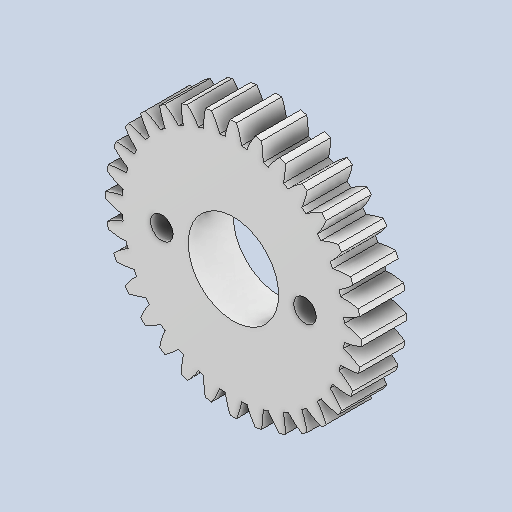
# Autodesk Inventor part: 平歯車1
Saved by Autodesk Inventor 2025.2 (Build 292293000, 293)
## iProperties
CustomPartVersion: 1
Created: 2025-01-07
Part Number: 平歯車1
Material: ABS プラスチック
Document SubType Name: Modeling
Designer: haruy
Categories: <?xml version="1.0" encoding="UTF-16"?> <MemberInstance><Categories><FamilyTemplate><FamilyTemplateParameter ValueType="xs:double" Id="1" ObjectReferenceKey="da_z" ObjectType="kUserParameterObject"/><FamilyTemplateParameter ValueType="xs:double" Id="2" ObjectReferenceKey="da_b" ObjectType="kUserParameterObject"/><FamilyTemplateParameter ValueType="xs:double" Id="3" ObjectReferenceKey="da_beta" ObjectType="kUserParameterObject"/><FamilyTemplateParameter ValueType="xs:double" Id="4" ObjectReferenceKey="da_da" ObjectType="kUserParameterObject"/><FamilyTemplateParameter ValueType="xs:double" Id="5" ObjectReferenceKey="da_aw" ObjectType="kUserParameterObject"/><FamilyTemplateParameter ValueType="xs:string" Id="6" ObjectReferenceKey="EAIAABAAAACIAQAAAAAAAIAAAAAAAAAA" ObjectType="83910656" SubObjectId="SurfaceGeometry"/></FamilyTemplate><ParamToTemplateMap><ParamToTemplate CategoryParameter="//CategoryParameter[@InternalName='046C89C9-8512-4d59-83FE-43B91F4F132A']" TemplateParameter="1"/><ParamToTemplate CategoryParameter="//CategoryParameter[@InternalName='2552DF32-E462-4b46-AEBF-C6C7768E72AC']" TemplateParameter="2"/><ParamToTemplate CategoryParameter="//CategoryParameter[@InternalName='C9EE641D-15FC-4fae-A226-E94C4372FDD7']" TemplateParameter="3"/><ParamToTemplate><ParamToTemplate CategoryParameter="//CategoryParameter[@InternalName='00B6519A-459B-49c7-AD84-2E56D39A5744']" ConstantValue="0.000000"/></ParamToTemplate><ParamToTemplate><ParamToTemplate CategoryParameter="//CategoryParameter[@InternalName='04B31F0E-C7A6-4894-AA32-9629BEFACF47']" ConstantValue="1.000000"/></ParamToTemplate><ParamToTemplate><ParamToTemplate CategoryParameter="//CategoryParameter[@InternalName='43CBEC2E-7847-49e7-A936-2F7889FCB2D9']" ConstantValue="0.250000"/></ParamToTemplate><ParamToTemplate><ParamToTemplate CategoryParameter="//CategoryParameter[@InternalName='B1EFC894-105D-4ebd-86BF-FA20ED196853']" ConstantValue="0.350000"/></ParamToTemplate><ParamToTemplate><ParamToTemplate CategoryParameter="//CategoryParameter[@InternalName='51175063-3D10-4879-93E8-6246FE8B403D']" ConstantValue="2060000000.000000"/></ParamToTemplate><ParamToTemplate><ParamToTemplate CategoryParameter="//CategoryParameter[@InternalName='A3A52E27-4454-46a9-B0BD-C932399B70AF']" ConstantValue="0.300000"/></ParamToTemplate><ParamToTemplate><ParamToTemplate CategoryParameter="//CategoryParameter[@InternalName='91B76062-C214-41d9-B1B9-14D2AB99603D']" ConstantValue="0.100000"/></ParamToTemplate><ParamToTemplate><ParamToTemplate CategoryParameter="//CategoryParameter[@InternalName='374E806E-8B8A-4dda-A9AA-1039D6500AD2']" ConstantValue="10.000000"/></ParamToTemplate><ParamToTemplate><ParamToTemplate CategoryParameter="//CategoryParameter[@InternalName='2D373A89-B862-43d6-8D0B-0CBF12AB9F6C']" ConstantValue="0.349066"/></ParamToTemplate><ParamToTemplate CategoryParameter="//CategoryParameter[@InternalName='37777632-D6A2-4fac-9D53-DB8ACD95C989']" TemplateParameter="4"/><ParamToTemplate CategoryParameter="//CategoryParameter[@InternalName='FD1017F1-B727-4f7e-9707-0F86F1FF9423']" TemplateParameter="5"/><ParamToTemplate><ParamToTemplate CategoryParameter="//CategoryParameter[@InternalName='9E1B4470-B2D3-4ff1-B813-535BB4CDF51A']" ConstantValue="3520000.000000"/></ParamToTemplate><ParamToTemplate><ParamToTemplate CategoryParameter="//CategoryParameter[@InternalName='F8452263-BFF6-458c-9FB1-07C4B99E95CD']" ConstantValue="11400000.000000"/></ParamToTemplate><ParamToTemplate><ParamToTemplate CategoryParameter="//CategoryParameter[@InternalName='3E3BB259-FD49-497f-8171-6EBC954A3479']" ConstantValue="2.000000"/></ParamToTemplate><ParamToTemplate CategoryParameter="//CategoryParameter[@InternalName='27C3BAF2-7550-4e4b-AE2C-0DB134B7D9B7']" TemplateParameter="6"/></ParamToTemplateMap><Category DisplayName="Gear" InternalName="DC85795E-93AB-48d5-8EEE-5A27447B64BD" Mnemonic="Gear"><CategoryParameter DisplayName="z" InternalName="046C89C9-8512-4d59-83FE-43B91F4F132A" Mnemonic="z"/><CategoryParameter DisplayName="b" InternalName="2552DF32-E462-4b46-AEBF-C6C7768E72AC" Mnemonic="b"/><CategoryParameter DisplayName="||b|" InternalName="C9EE641D-15FC-4fae-A226-E94C4372FDD7" Mnemonic="beta"/><CategoryParameter DisplayName="x" InternalName="00B6519A-459B-49c7-AD84-2E56D39A5744" Mnemonic="x"/><CategoryParameter DisplayName="a*" InternalName="04B31F0E-C7A6-4894-AA32-9629BEFACF47" Mnemonic="a"/><CategoryParameter DisplayName="c*" InternalName="43CBEC2E-7847-49e7-A936-2F7889FCB2D9" Mnemonic="c"/><CategoryParameter DisplayName="r|.f|*" InternalName="B1EFC894-105D-4ebd-86BF-FA20ED196853" Mnemonic="rf"/><CategoryParameter DisplayName="E" InternalName="51175063-3D10-4879-93E8-6246FE8B403D" Mnemonic="E"/><CategoryParameter DisplayName="||m|" InternalName="A3A52E27-4454-46a9-B0BD-C932399B70AF" Mnemonic="mi"/><Category DisplayName="SpurGear" InternalName="26C5A22E-A91E-4dfd-A3B3-23CCAFAE1764" Mnemonic="SpurGear"><CategoryParameter DisplayName="m" InternalName="91B76062-C214-41d9-B1B9-14D2AB99603D" Mnemonic="m"/><CategoryParameter DisplayName="P" InternalName="374E806E-8B8A-4dda-A9AA-1039D6500AD2" Mnemonic="PP"/><CategoryParameter DisplayName="||a|" InternalName="2D373A89-B862-43d6-8D0B-0CBF12AB9F6C" Mnemonic="alpha"/><CategoryParameter DisplayName="d|.a|" InternalName="37777632-D6A2-4fac-9D53-DB8ACD95C989" Mnemonic="da"/><CategoryParameter DisplayName="a|.w|" InternalName="FD1017F1-B727-4f7e-9707-0F86F1FF9423" Mnemonic="aw"/><CategoryParameter DisplayName="||s||.Flim|" InternalName="9E1B4470-B2D3-4ff1-B813-535BB4CDF51A" Mnemonic="sFlim"/><CategoryParameter DisplayName="||s||.Hlim|" InternalName="F8452263-BFF6-458c-9FB1-07C4B99E95CD" Mnemonic="sHlim"/><CategoryParameter DisplayName="タイプ" InternalName="3E3BB259-FD49-497f-8171-6EBC954A3479" Mnemonic="type"/><CategoryParameter DisplayName="PitchDiameter" InternalName="27C3BAF2-7550-4e4b-AE2C-0DB134B7D9B7" Mnemonic="IDS_PITCHDIAM"/></Category></Category></Categories></MemberInstance>
Density: 1.06 g/cm^3
Appearance: 滑らか - 白
Mass: 37.6143 g
Surface Area: 28.126 cm^2
Volume: 4.79163 cm^3
Author: haruy
Autodesk Inventor part; units mm, degrees
sketch "Sketch1" plane through (0, 0, 0) normal (0, 0, 1) x (1, 0, 0)
  circle A0 centre (0, 0) radius 17
  dimension "d0" = 34
  constraints: 1 centre point
  measures "d0" diameter of A0
extrude "Extrusion1" add sketch "Sketch1" along normal blind 6
ref_plane "Work Plane2" through (0, 0, 3) normal (0, 0, 1) x (1, 0, 0)
sketch "Sketch2" plane through (0, 0, 0) normal (0, 0, -1) x (-1, 0, 0)
  circle A0 centre (0, 0) radius 17 projected
  circle A1 centre (0, 0) radius 16
  dimension "d3" = 32
  constraints: 1 centre point, 1 coincident
  measures "d3" diameter of A1
surface extrude "ピッチ円直径" sketch "Sketch2" against normal through all shown no curves A1
ref_plane "Work Plane8" through (0, 0, 0) normal (0.9951847, 0.0980171, 0) x (0, 0, 1)
ref_plane "Work Plane9" through (0, 0, 0) normal (1, 0, 0) x (0, 1, 0)
spur gear teeth "平歯車" teeth 32 pitch diameter 32 tip diameter 34 root diameter 29.5 face width 6 start plane through (0, 0, 0) normal (0, 0, -1) x (-1, 0, 0)
sketch "スケッチ3" plane through (0, 0, 6) normal (0, 0, 1) x (1, 0, 0)
  circle A0 centre (0, 0) radius 6
  circle A1 centre (0, 0) radius 9.5
  circle A2 centre (-9.5, 0) radius 1.5
  circle A3 centre (9.5, 0) radius 1.5
  dimension "d50" = 19
  dimension "d49" = 12
  dimension "d51" = 3
  dimension "d54" = 360
  constraints: 3 centre point, 2 coincident, 1 horizontal alignment, 7 other
  measures "d49" diameter of A0
  measures "d51" diameter of A2
extrude "押し出し2" cut sketch "スケッチ3" against normal blind 10 contours A0 | A1 A3 | A1 A3 | A2 A1 | A1 A2
sketch "スケッチ4" plane through (0, 0, 6) normal (0, 0, 1) x (1, 0, 0)
  circle A0 centre (9.5, 0) radius 1.5 projected
  circle A1 centre (-9.5, 0) radius 1.5 projected
  circle A2 centre (0, 0) radius 6 projected
  arc A3 (-3.7247, 16.5869) -> (-3.934, 14.2157) centre (6.3329, 14.5044) ccw projected
  arc A4 (-3.934, 14.2157) -> (-4.6268, 14.0055) centre (0, 0) ccw projected
  arc A5 (-4.6268, 14.0055) -> (-6.1182, 15.8609) centre (-13.3238, 8.5416) ccw projected
  arc A6 (-6.1182, 15.8609) -> (-6.8891, 15.5416) centre (0, 0) ccw projected
  arc A7 (-6.8891, 15.5416) -> (-6.6318, 13.1751) centre (3.3815, 15.4612) ccw projected
  arc A8 (-6.6318, 13.1751) -> (-7.2702, 12.8338) centre (0, 0) ccw projected
  arc A9 (-7.2702, 12.8338) -> (-9.095, 14.3625) centre (-14.7342, 5.7781) ccw projected
  arc A10 (-9.095, 14.3625) -> (-9.7887, 13.8989) centre (0, 0) ccw projected
  arc A11 (-9.7887, 13.8989) -> (-9.0747, 11.6281) centre (0.3002, 15.8238) ccw projected
  arc A12 (-9.0747, 11.6281) -> (-9.6343, 11.1688) centre (0, 0) ccw projected
  arc A13 (-9.6343, 11.1688) -> (-11.7222, 12.3122) centre (-15.5783, 2.7926) ccw projected
  arc A14 (-11.7222, 12.3122) -> (-12.3122, 11.7222) centre (0, 0) ccw projected
  arc A15 (-12.3122, 11.7222) -> (-11.1688, 9.6343) centre (-2.7926, 15.5783) ccw projected
  arc A16 (-11.1688, 9.6343) -> (-11.6281, 9.0747) centre (0, 0) ccw projected
  arc A17 (-11.6281, 9.0747) -> (-13.8989, 9.7887) centre (-15.8238, -0.3002) ccw projected
  arc A18 (-13.8989, 9.7887) -> (-14.3625, 9.095) centre (0, 0) ccw projected
  arc A19 (-14.3625, 9.095) -> (-12.8338, 7.2702) centre (-5.7781, 14.7342) ccw projected
  arc A20 (-12.8338, 7.2702) -> (-13.1751, 6.6318) centre (0, 0) ccw projected
  arc A21 (-13.1751, 6.6318) -> (-15.5416, 6.8891) centre (-15.4612, -3.3815) ccw projected
  arc A22 (-15.5416, 6.8891) -> (-15.8609, 6.1182) centre (0, 0) ccw projected
  arc A23 (-15.8609, 6.1182) -> (-14.0055, 4.6268) centre (-8.5416, 13.3238) ccw projected
  arc A24 (-14.0055, 4.6268) -> (-14.2157, 3.934) centre (0, 0) ccw projected
  arc A25 (-14.2157, 3.934) -> (-16.5869, 3.7247) centre (-14.5044, -6.3329) ccw projected
  arc A26 (-16.5869, 3.7247) -> (-16.7497, 2.9064) centre (0, 0) ccw projected
  arc A27 (-16.7497, 2.9064) -> (-14.6391, 1.8056) centre (-10.9768, 11.4014) ccw projected
  arc A28 (-14.6391, 1.8056) -> (-14.71, 1.0851) centre (0, 0) ccw projected
  arc A29 (-14.71, 1.0851) -> (-16.9949, 0.4172) centre (-12.9902, -9.0408) ccw projected
  arc A30 (-16.9949, 0.4172) -> (-16.9949, -0.4172) centre (0, 0) ccw projected
  arc A31 (-16.9949, -0.4172) -> (-14.71, -1.0851) centre (-12.9902, 9.0408) ccw projected
  arc A32 (-14.71, -1.0851) -> (-14.6391, -1.8056) centre (0, 0) ccw projected
  arc A33 (-14.6391, -1.8056) -> (-16.7497, -2.9064) centre (-10.9768, -11.4014) ccw projected
  arc A34 (-16.7497, -2.9064) -> (-16.5869, -3.7247) centre (0, 0) ccw projected
  arc A35 (-16.5869, -3.7247) -> (-14.2157, -3.934) centre (-14.5044, 6.3329) ccw projected
  arc A36 (-14.2157, -3.934) -> (-14.0055, -4.6268) centre (0, 0) ccw projected
  arc A37 (-14.0055, -4.6268) -> (-15.8609, -6.1182) centre (-8.5416, -13.3238) ccw projected
  arc A38 (-15.8609, -6.1182) -> (-15.5416, -6.8891) centre (0, 0) ccw projected
  arc A39 (-15.5416, -6.8891) -> (-13.1751, -6.6318) centre (-15.4612, 3.3815) ccw projected
  arc A40 (-13.1751, -6.6318) -> (-12.8338, -7.2702) centre (0, 0) ccw projected
  arc A41 (-12.8338, -7.2702) -> (-14.3625, -9.095) centre (-5.7781, -14.7342) ccw projected
  arc A42 (-14.3625, -9.095) -> (-13.8989, -9.7887) centre (0, 0) ccw projected
  arc A43 (-13.8989, -9.7887) -> (-11.6281, -9.0747) centre (-15.8238, 0.3002) ccw projected
  arc A44 (-11.6281, -9.0747) -> (-11.1688, -9.6343) centre (0, 0) ccw projected
  arc A45 (-11.1688, -9.6343) -> (-12.3122, -11.7222) centre (-2.7926, -15.5783) ccw projected
  arc A46 (-12.3122, -11.7222) -> (-11.7222, -12.3122) centre (0, 0) ccw projected
  arc A47 (-11.7222, -12.3122) -> (-9.6343, -11.1688) centre (-15.5783, -2.7926) ccw projected
  arc A48 (-9.6343, -11.1688) -> (-9.0747, -11.6281) centre (0, 0) ccw projected
  arc A49 (-9.0747, -11.6281) -> (-9.7887, -13.8989) centre (0.3002, -15.8238) ccw projected
  arc A50 (-9.7887, -13.8989) -> (-9.095, -14.3625) centre (0, 0) ccw projected
  arc A51 (-9.095, -14.3625) -> (-7.2702, -12.8338) centre (-14.7342, -5.7781) ccw projected
  arc A52 (-7.2702, -12.8338) -> (-6.6318, -13.1751) centre (0, 0) ccw projected
  arc A53 (-6.6318, -13.1751) -> (-6.8891, -15.5416) centre (3.3815, -15.4612) ccw projected
  arc A54 (-6.8891, -15.5416) -> (-6.1182, -15.8609) centre (0, 0) ccw projected
  arc A55 (-6.1182, -15.8609) -> (-4.6268, -14.0055) centre (-13.3238, -8.5416) ccw projected
  arc A56 (-4.6268, -14.0055) -> (-3.934, -14.2157) centre (0, 0) ccw projected
  arc A57 (-3.934, -14.2157) -> (-3.7247, -16.5869) centre (6.3329, -14.5044) ccw projected
  arc A58 (-3.7247, -16.5869) -> (-2.9064, -16.7497) centre (0, 0) ccw projected
  arc A59 (-2.9064, -16.7497) -> (-1.8056, -14.6391) centre (-11.4014, -10.9768) ccw projected
  arc A60 (-1.8056, -14.6391) -> (-1.0851, -14.71) centre (0, 0) ccw projected
  arc A61 (-1.0851, -14.71) -> (-0.4172, -16.9949) centre (9.0408, -12.9902) ccw projected
  arc A62 (-0.4172, -16.9949) -> (0.4172, -16.9949) centre (0, 0) ccw projected
  arc A63 (0.4172, -16.9949) -> (1.0851, -14.71) centre (-9.0408, -12.9902) ccw projected
  arc A64 (1.0851, -14.71) -> (1.8056, -14.6391) centre (0, 0) ccw projected
  arc A65 (1.8056, -14.6391) -> (2.9064, -16.7497) centre (11.4014, -10.9768) ccw projected
  arc A66 (2.9064, -16.7497) -> (3.7247, -16.5869) centre (0, 0) ccw projected
  arc A67 (3.7247, -16.5869) -> (3.934, -14.2157) centre (-6.3329, -14.5044) ccw projected
  arc A68 (3.934, -14.2157) -> (4.6268, -14.0055) centre (0, 0) ccw projected
  arc A69 (4.6268, -14.0055) -> (6.1182, -15.8609) centre (13.3238, -8.5416) ccw projected
  arc A70 (6.1182, -15.8609) -> (6.8891, -15.5416) centre (0, 0) ccw projected
  arc A71 (6.8891, -15.5416) -> (6.6318, -13.1751) centre (-3.3815, -15.4612) ccw projected
  arc A72 (6.6318, -13.1751) -> (7.2702, -12.8338) centre (0, 0) ccw projected
  arc A73 (7.2702, -12.8338) -> (9.095, -14.3625) centre (14.7342, -5.7781) ccw projected
  arc A74 (9.095, -14.3625) -> (9.7887, -13.8989) centre (0, 0) ccw projected
  arc A75 (9.7887, -13.8989) -> (9.0747, -11.6281) centre (-0.3002, -15.8238) ccw projected
  arc A76 (9.0747, -11.6281) -> (9.6343, -11.1688) centre (0, 0) ccw projected
  arc A77 (9.6343, -11.1688) -> (11.7222, -12.3122) centre (15.5783, -2.7926) ccw projected
  arc A78 (11.7222, -12.3122) -> (12.3122, -11.7222) centre (0, 0) ccw projected
  arc A79 (12.3122, -11.7222) -> (11.1688, -9.6343) centre (2.7926, -15.5783) ccw projected
  arc A80 (11.1688, -9.6343) -> (11.6281, -9.0747) centre (0, 0) ccw projected
  arc A81 (11.6281, -9.0747) -> (13.8989, -9.7887) centre (15.8238, 0.3002) ccw projected
  arc A82 (13.8989, -9.7887) -> (14.3625, -9.095) centre (0, 0) ccw projected
  arc A83 (14.3625, -9.095) -> (12.8338, -7.2702) centre (5.7781, -14.7342) ccw projected
  arc A84 (12.8338, -7.2702) -> (13.1751, -6.6318) centre (0, 0) ccw projected
  arc A85 (13.1751, -6.6318) -> (15.5416, -6.8891) centre (15.4612, 3.3815) ccw projected
  arc A86 (15.5416, -6.8891) -> (15.8609, -6.1182) centre (0, 0) ccw projected
  arc A87 (15.8609, -6.1182) -> (14.0055, -4.6268) centre (8.5416, -13.3238) ccw projected
  arc A88 (14.0055, -4.6268) -> (14.2157, -3.934) centre (0, 0) ccw projected
  arc A89 (14.2157, -3.934) -> (16.5869, -3.7247) centre (14.5044, 6.3329) ccw projected
  arc A90 (16.5869, -3.7247) -> (16.7497, -2.9064) centre (0, 0) ccw projected
  arc A91 (16.7497, -2.9064) -> (14.6391, -1.8056) centre (10.9768, -11.4014) ccw projected
  arc A92 (14.6391, -1.8056) -> (14.71, -1.0851) centre (0, 0) ccw projected
  arc A93 (14.71, -1.0851) -> (16.9949, -0.4172) centre (12.9902, 9.0408) ccw projected
  arc A94 (16.9949, -0.4172) -> (16.9949, 0.4172) centre (0, 0) ccw projected
  arc A95 (16.9949, 0.4172) -> (14.71, 1.0851) centre (12.9902, -9.0408) ccw projected
  arc A96 (14.71, 1.0851) -> (14.6391, 1.8056) centre (0, 0) ccw projected
  arc A97 (14.6391, 1.8056) -> (16.7497, 2.9064) centre (10.9768, 11.4014) ccw projected
  arc A98 (16.7497, 2.9064) -> (16.5869, 3.7247) centre (0, 0) ccw projected
  arc A99 (16.5869, 3.7247) -> (14.2157, 3.934) centre (14.5044, -6.3329) ccw projected
  arc A100 (14.2157, 3.934) -> (14.0055, 4.6268) centre (0, 0) ccw projected
  arc A101 (14.0055, 4.6268) -> (15.8609, 6.1182) centre (8.5416, 13.3238) ccw projected
  arc A102 (15.8609, 6.1182) -> (15.5416, 6.8891) centre (0, 0) ccw projected
  arc A103 (15.5416, 6.8891) -> (13.1751, 6.6318) centre (15.4612, -3.3815) ccw projected
  arc A104 (13.1751, 6.6318) -> (12.8338, 7.2702) centre (0, 0) ccw projected
  arc A105 (12.8338, 7.2702) -> (14.3625, 9.095) centre (5.7781, 14.7342) ccw projected
  arc A106 (14.3625, 9.095) -> (13.8989, 9.7887) centre (0, 0) ccw projected
  arc A107 (13.8989, 9.7887) -> (11.6281, 9.0747) centre (15.8238, -0.3002) ccw projected
  arc A108 (11.6281, 9.0747) -> (11.1688, 9.6343) centre (0, 0) ccw projected
  arc A109 (11.1688, 9.6343) -> (12.3122, 11.7222) centre (2.7926, 15.5783) ccw projected
  arc A110 (12.3122, 11.7222) -> (11.7222, 12.3122) centre (0, 0) ccw projected
  arc A111 (11.7222, 12.3122) -> (9.6343, 11.1688) centre (15.5783, 2.7926) ccw projected
  arc A112 (9.6343, 11.1688) -> (9.0747, 11.6281) centre (0, 0) ccw projected
  arc A113 (9.0747, 11.6281) -> (9.7887, 13.8989) centre (-0.3002, 15.8238) ccw projected
  arc A114 (9.7887, 13.8989) -> (9.095, 14.3625) centre (0, 0) ccw projected
  arc A115 (9.095, 14.3625) -> (7.2702, 12.8338) centre (14.7342, 5.7781) ccw projected
  arc A116 (7.2702, 12.8338) -> (6.6318, 13.1751) centre (0, 0) ccw projected
  arc A117 (6.6318, 13.1751) -> (6.8891, 15.5416) centre (-3.3815, 15.4612) ccw projected
  arc A118 (6.8891, 15.5416) -> (6.1182, 15.8609) centre (0, 0) ccw projected
  arc A119 (6.1182, 15.8609) -> (4.6268, 14.0055) centre (13.3238, 8.5416) ccw projected
  arc A120 (4.6268, 14.0055) -> (3.934, 14.2157) centre (0, 0) ccw projected
  arc A121 (3.934, 14.2157) -> (3.7247, 16.5869) centre (-6.3329, 14.5044) ccw projected
  arc A122 (3.7247, 16.5869) -> (2.9064, 16.7497) centre (0, 0) ccw projected
  arc A123 (2.9064, 16.7497) -> (1.8056, 14.6391) centre (11.4014, 10.9768) ccw projected
  arc A124 (1.8056, 14.6391) -> (1.0851, 14.71) centre (0, 0) ccw projected
  arc A125 (1.0851, 14.71) -> (0.4172, 16.9949) centre (-9.0408, 12.9902) ccw projected
  arc A126 (0.4172, 16.9949) -> (-0.4172, 16.9949) centre (0, 0) ccw projected
  arc A127 (-0.4172, 16.9949) -> (-1.0851, 14.71) centre (9.0408, 12.9902) ccw projected
  arc A128 (-1.0851, 14.71) -> (-1.8056, 14.6391) centre (0, 0) ccw projected
  arc A129 (-1.8056, 14.6391) -> (-2.9064, 16.7497) centre (-11.4014, 10.9768) ccw projected
  arc A130 (-2.9064, 16.7497) -> (-3.7247, 16.5869) centre (0, 0) ccw projected
equation "\"d0\" = da_da"
equation "\"d1\" = da_b"
equation "\"d3\" = da_d"
equation "\"d16\" = da_aw"
equation "\"d43\" = da_aw"
equation "\"d46\" = da_aw"
equation "\"da_da\" = 34"
equation "\"da_b\" = 6"
equation "\"da_d\" = 32"
equation "\"da_aw\" = 32"
body "Solid1"
body "Srf1"
